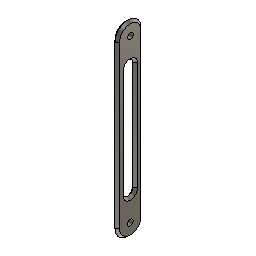
intermediate_arm_part_Asheeyana_Ahmed (Autodesk Fusion 360 design; units mm, degrees)
Autodesk Fusion 360 part; units mm, degrees
note: some values were not read from the file. Set by a fixed rule: which sketch regions a step uses.
sketch "Sketch1" plane through (0, 0, 0) normal (1, 0, 0) x (0, 1, 0)
  line L0 (2.8, 6) -> (2.8, 5.1079)
  arc A0 (2.8, 6) -> (-2.8, 6) centre (0, 6) ccw
  arc A1 (-2.8, 5.1079) -> (2.8, 5.1079) centre (0, 0) ccw
  line L1 (-2.8, 5.1079) -> (-2.8, 6)
  circle A2 centre (0, 0) radius 2.5
  circle A3 centre (0, 0) radius 11.25
  circle A4 centre (0, 0) radius 2.5
  line L2 (2.8, 6) -> (2.8, 5.1079)
  circle A5 centre (0, 0) radius 11.25
  line L3 (-2.8, 5.1079) -> (-2.8, 6)
  arc A6 (2.8, 6) -> (-2.8, 6) centre (0, 6) ccw
  arc A7 (-2.8, 5.1079) -> (2.8, 5.1079) centre (0, 0) ccw
  arc A8 (-2.8, 144.8079) -> (2.8, 144.8079) centre (0, 139.7) ccw
  line L4 (2.8, 145.7) -> (2.8, 144.8079)
  circle A9 centre (0, 139.7) radius 11.25
  circle A10 centre (0, 139.7) radius 11.25
  circle A11 centre (0, 139.7) radius 2.5
  line L5 (-2.8, 144.8079) -> (-2.8, 145.7)
  line L6 (2.8, 145.7) -> (2.8, 144.8079)
  circle A12 centre (0, 139.7) radius 2.5
  arc A13 (2.8, 145.7) -> (-2.8, 145.7) centre (0, 145.7) ccw
  arc A14 (2.8, 145.7) -> (-2.8, 145.7) centre (0, 145.7) ccw
  line L7 (-2.8, 144.8079) -> (-2.8, 145.7)
  arc A15 (-2.8, 144.8079) -> (2.8, 144.8079) centre (0, 139.7) ccw
  line L8 (0, 139.7) -> (0, 0) construction
  line L9 (0, 139.7) -> (-11.25, 139.7) construction
  line L10 (0, 0) -> (-11.25, 0) construction
  line L11 (0, 69.85) -> (50, 69.85) construction
  arc A16 (-7.2247, 139.7) -> (-7.2753, 140.1491) centre (-629.3846, 69.85) ccw
  arc A17 (-7.2753, -0.4491) -> (-7.2247, 0) centre (-629.3846, 69.85) ccw
  line L12 (11.25, 139.7) -> (11.25, 0)
  line L13 (-11.25, 139.7) -> (-11.25, 0)
  arc A18 (7.25, 116.7) -> (-7.25, 116.7) centre (0, 116.7) ccw
  arc A19 (-7.25, 23) -> (7.25, 23) centre (0, 23) ccw
  line L14 (-7.25, 116.7) -> (-7.25, 23)
  line L15 (7.25, 116.7) -> (7.25, 23)
  circle A20 centre (0, 128.45) radius 2.25
  circle A21 centre (0, 11.25) radius 2.25
  arc A22 (-4.25, 23) -> (4.25, 23) centre (0, 23) ccw
  line L16 (4.25, 116.7) -> (4.25, 23)
  arc A23 (4.25, 116.7) -> (-4.25, 116.7) centre (0, 116.7) ccw
  line L17 (-4.25, 116.7) -> (-4.25, 23)
  point P0 (0, 5.375)
  point P1 (0, 5.375)
  point P2 (0, 150.95)
  point P3 (0, 145.075)
  point P4 (0, 150.95)
  point P5 (0, 139.7)
  point P6 (0, 139.7)
  point P7 (0, 145.075)
  dimension "d1" = 11.65
  dimension "d3" = 5.6
  dimension "d4" = 6
  dimension "d5" = 5
  dimension "d6" = 22.5
  dimension "d8" = 11.65
  dimension "d9" = 5.6
  dimension "d10" = 6
  dimension "d11" = 5
  dimension "d12" = 22.5
  dimension "d14" = 11.65
  dimension "d15" = 5.6
  dimension "d16" = 6
  dimension "d17" = 5
  dimension "d18" = 22.5
  dimension "d19" = 11.65
  dimension "d20" = 5.6
  dimension "d21" = 6
  dimension "d22" = 5
  dimension "d23" = 22.5
  dimension "d60" = 4.5
  dimension "d63" = -3
  constraint tangent L0 A0
  constraint tangent A0 L1
  constraint concentric A1 A2
  constraint concentric A2 A3
  constraint tangent L2 A6
  constraint tangent L3 A6
  constraint concentric A4 A7
  constraint concentric A4 A5
  constraint tangent L6 A14
  constraint tangent A14 L7
  constraint concentric A8 A11
  constraint concentric A9 A11
  constraint coincident P4 A9
  constraint tangent L4 A13
  constraint tangent L5 A13
  constraint concentric A12 A15
  constraint concentric A10 A12
  constraint coincident P4 A10
  constraint coincident P6 P5
  constraint coincident A1.centre A2.centre
  constraint vertical L8
  constraint horizontal L9
  constraint coincident A5 L10.end
  constraint perpendicular L8 L10
  constraint midpoint L8 L11.start
  constraint perpendicular L8 L11
  constraint coincident L9 A16.start
  constraint concentric A16 A17
  constraint coincident L10 A17.end
  constraint tangent A5 L12
  constraint tangent A3 L13
  constraint coincident L8 A20.centre
  constraint coincident A9 A20.centre
  constraint symmetric L11 A20 A21
  measures "d1" diameter of A1
  measures "d3" diameter of A0
  measures "d4" distance of A1.centre A0.centre
  measures "d5" diameter of A2
  measures "d6" diameter of A3
  measures "d8" diameter of A7
  measures "d9" diameter of A6
  measures "d10" distance of A0.centre A1.centre
  measures "d11" diameter of A4
  measures "d12" diameter of A5
  measures "d14" diameter of A8
  measures "d15" diameter of A14
  measures "d16" distance of A13.centre P6
  measures "d17" diameter of A11
  measures "d18" diameter of A9
  measures "d19" diameter of A15
  measures "d20" diameter of A13
  measures "d21" distance of P6 A13.centre
  measures "d22" diameter of A12
  measures "d23" diameter of A10
  measures "d60" diameter of A20
extrude "Extrude1" add sketch "Sketch1" against normal blind 4 contours L0 A0 A1 L1 L2 L3 A6 A7 | A3 A5 A21 | A3 A5 A9 A10 L12 L13 A20 A21 | A3 A5 A21 | A3 A5 A21 | A9 A10 A20 | A9 A10 A20 | A9 A10 A20 | A8 L4 L5 L6 A13 A14 L7 A15 | A18 A19 L14 L15
ref_plane "WorkPlane1" through (25.5, 0, 69.85) normal (1, 0, 0) x (0, 1, 0)
chamfer "Chamfer1" distance 2 angle 45 8 edges at (0, 11.25, 69.85) (0, 0, -11.25) (0, -11.25, 69.85) (0, 0, 150.95) (-4, 0, 150.95) (-4, 11.25, 69.85) (-4, 0, -11.25) (-4, -11.25, 69.85)
chamfer "Chamfer3" distance 2 angle 45 8 edges at (0, 0, 120.95) (0, 4.25, 69.85) (0, 0, 18.75) (0, -4.25, 69.85) (-4, 0, 120.95) (-4, -4.25, 69.85) (-4, 0, 18.75) (-4, 4.25, 69.85)
sketch "Sketch2" plane through (25.5, 0, 0) normal (1, 0, 0) x (0, 1, 0)
  arc A0 (-2.8, 144.8079) -> (2.8, 144.8079) centre (0, 139.7) ccw
  arc A1 (2.8, 145.7) -> (-2.8, 145.7) centre (0, 145.7) ccw
  line L0 (11.25, 139.7) -> (11.25, 0)
  line L1 (0, 139.7) -> (0, 0) construction
  circle A2 centre (0, 139.7) radius 11.25
  line L2 (-2.8, 144.8079) -> (-2.8, 145.7)
  circle A3 centre (0, 139.7) radius 11.25
  line L3 (-11.25, 139.7) -> (-11.25, 0)
  circle A4 centre (0, 0) radius 11.25
  line L4 (2.8, 145.7) -> (2.8, 144.8079)
  circle A5 centre (0, 139.7) radius 2.5
  line L5 (0, 139.7) -> (-11.25, 139.7) construction
  line L6 (2.8, 145.7) -> (2.8, 144.8079)
  arc A6 (7.25, 116.7) -> (-7.25, 116.7) centre (0, 116.7) ccw
  circle A7 centre (0, 139.7) radius 2.5
  arc A8 (-7.2247, 139.7) -> (-7.2753, 140.1491) centre (-629.3846, 69.85) ccw
  arc A9 (2.8, 145.7) -> (-2.8, 145.7) centre (0, 145.7) ccw
  line L7 (-2.8, 144.8079) -> (-2.8, 145.7)
  line L8 (-7.25, 116.7) -> (-7.25, 23)
  line L9 (7.25, 116.7) -> (7.25, 23)
  arc A10 (-2.8, 144.8079) -> (2.8, 144.8079) centre (0, 139.7) ccw
  circle A11 centre (0, 0) radius 2.5
  arc A12 (2.8, 6) -> (-2.8, 6) centre (0, 6) ccw
  arc A13 (2.8, 6) -> (-2.8, 6) centre (0, 6) ccw
  line L10 (-2.8, 5.1079) -> (-2.8, 6)
  line L11 (2.8, 6) -> (2.8, 5.1079)
  circle A14 centre (0, 0) radius 2.5
  arc A15 (-2.8, 5.1079) -> (2.8, 5.1079) centre (0, 0) ccw
  arc A16 (-2.8, 5.1079) -> (2.8, 5.1079) centre (0, 0) ccw
  line L12 (2.8, 6) -> (2.8, 5.1079)
  arc A17 (-7.25, 23) -> (7.25, 23) centre (0, 23) ccw
  arc A18 (-7.2753, -0.4491) -> (-7.2247, 0) centre (-629.3846, 69.85) ccw
  circle A19 centre (0, 0) radius 11.25
  line L13 (0, 0) -> (-11.25, 0) construction
  line L14 (-2.8, 5.1079) -> (-2.8, 6)
  point P0 (0, 69.85)
  point P1 (0, 150.95)
  point P2 (0, 139.7)
  point P3 (0, 145.075)
  point P4 (0, 150.95)
  point P5 (0, 5.375)
  point P6 (0, 145.075)
  point P7 (0, 139.7)
  point P8 (0, 5.375)
  dimension "d36" = 11.65
  dimension "d37" = 5.6
  dimension "d38" = 6
  dimension "d39" = 5
  dimension "d40" = 22.5
  dimension "d41" = 11.65
  dimension "d42" = 5.6
  dimension "d43" = 6
  dimension "d44" = 5
  dimension "d45" = 22.5
  dimension "d46" = 11.65
  dimension "d47" = 5.6
  dimension "d48" = 6
  dimension "d49" = 5
  dimension "d50" = 22.5
  dimension "d51" = 11.65
  dimension "d52" = 5.6
  dimension "d53" = 6
  dimension "d54" = 5
  dimension "d55" = 22.5
  dimension "d56" = 4
  dimension "d57" = 4
  constraint tangent A12 L12
  constraint tangent A12 L10
  constraint concentric A11 A16
  constraint concentric A11 A19
  constraint tangent A13 L11
  constraint tangent A13 L14
  constraint concentric A14 A15
  constraint concentric A4 A14
  constraint tangent L4 A9
  constraint tangent A9 L7
  constraint concentric A0 A7
  constraint concentric A3 A7
  constraint coincident P4 A3
  constraint tangent A1 L6
  constraint tangent A1 L2
  constraint concentric A5 A10
  constraint concentric A2 A5
  constraint coincident P4 A2
  constraint coincident P7 P2
  constraint coincident L1.end A4.centre
  constraint vertical L1
  constraint horizontal L5
  constraint coincident P7 A0.centre
  constraint coincident L3.end A4
  constraint perpendicular L1 L13
  constraint midpoint P0 L1
  constraint coincident A8.start L5
  constraint concentric A8 A18
  constraint coincident A18.end L13
  constraint tangent L0 A4
  constraint tangent L3 A19
  measures "d36" diameter of A16
  measures "d37" diameter of A12
  measures "d38" distance of A12.centre L1.end
  measures "d39" diameter of A11
  measures "d40" diameter of A19
  measures "d41" diameter of A15
  measures "d42" diameter of A13
  measures "d43" distance of L1.end A12.centre
  measures "d44" diameter of A14
  measures "d45" diameter of A4
  measures "d46" diameter of A0
  measures "d47" diameter of A9
  measures "d48" distance of A1.centre P7
  measures "d49" diameter of A7
  measures "d50" diameter of A3
  measures "d51" diameter of A10
  measures "d52" diameter of A1
  measures "d53" distance of A1.centre P7
  measures "d54" diameter of A5
  measures "d55" diameter of A2
  measures "d56" distance of L3 L8
  measures "d57" distance of L0 L9
extrude "Extrude2" [suppressed]
